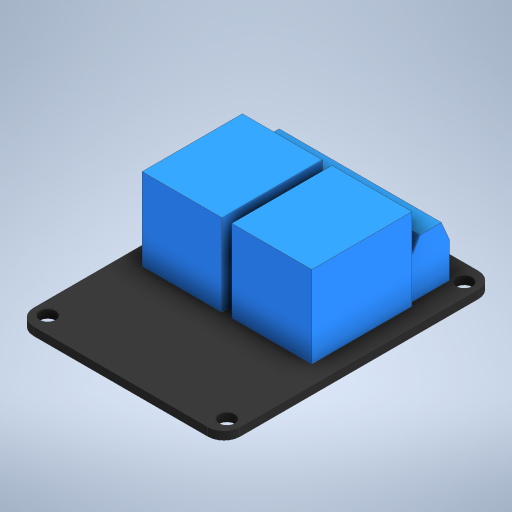
# Autodesk Inventor part: 더블 릴레이 모듈
Saved by Autodesk Inventor 2023.1 (Build 271208000, 208)
## iProperties
Created: 2022-08-14
Part Number: 더블 릴레이 모듈
Material: 일반
Document SubType Name: Modeling
Designer: fly01
Density: 1 g/cm^3
Appearance: 기본값
Author: fly01
Autodesk Inventor part; units mm, degrees
ref_plane "YZ Plane" through (0, 0, 0) normal (1, 0, 0) x (0, 1, 0)
ref_plane "XZ Plane" through (0, 0, 0) normal (0, 1, 0) x (-1, 0, 0)
ref_plane "XY Plane" through (0, 0, 0) normal (0, 0, 1) x (1, 0, 0)
sketch "스케치1" plane through (0, 0, 0) normal (0, 0, 1) x (1, 0, 0)
  point P0 (0, 0)
sketch "스케치2" plane through (0, 0, 0) normal (0, 1, 0) x (-1, 0, 0)
  line L0 (-16.35, -25.35) -> (16.35, -25.35)
  line L1 (19.35, -22.35) -> (19.35, 22.35)
  line L2 (16.35, 25.35) -> (-16.35, 25.35)
  line L3 (-19.35, 22.35) -> (-19.35, -22.35)
  line L4 (-19.35, -25.35) -> (19.35, 25.35) construction
  line L5 (19.35, -25.35) -> (-19.35, 25.35) construction
  circle A0 centre (16.8, 22.25) radius 1.5
  line L6 (0, 0) -> (0, -6.2498)
  line L7 (0, 0) -> (4.685, 0)
  circle A1 centre (16.8, -22.25) radius 1.5
  circle A2 centre (-16.8, 22.25) radius 1.5
  circle A3 centre (-16.8, -22.25) radius 1.5
  arc A4 (19.35, 22.35) -> (16.35, 25.35) centre (16.35, 22.35) ccw
  arc A5 (16.35, -25.35) -> (19.35, -22.35) centre (16.35, -22.35) ccw
  arc A6 (-19.35, -22.35) -> (-16.35, -25.35) centre (-16.35, -22.35) ccw
  arc A7 (-16.35, 25.35) -> (-19.35, 22.35) centre (-16.35, 22.35) ccw
  dimension "d0" = 38.7
  dimension "d1" = 50.7
  dimension "d2" = 3
  dimension "d3" = 30.6
  dimension "d4" = 44.5
  dimension "d5" = 3
  constraints: 16 end point, 8 centre point, 8 point on circle, 8 point on line, 8 tangent, 3 equal radius, 3 symmetric about line, 2 horizontal, 2 midpoint, 2 parallel, 1 perpendicular, 1 vertical, 3 other
  measures "d0" distance of L5.end L4.end
  measures "d1" distance of L4.end L5.start
  measures "d2" diameter of A0
  measures "d4" distance of A3.centre A2.centre
  measures "d5" radius of A4
extrude "돌출1" add sketch "스케치2" along normal blind 1.55
sketch "스케치3" plane through (0, 1.55, 0) normal (0, 1, 0) x (1, 0, 0)
  line L0 (-15.9, -5.45) -> (-0.9, -5.45)
  line L1 (-0.9, -5.45) -> (-0.9, 13.35)
  line L2 (-0.9, 13.35) -> (-15.9, 13.35)
  line L3 (-15.9, 13.35) -> (-15.9, -5.45)
  line L4 (-15.9, -5.45) -> (-0.9, 13.35) construction
  line L5 (-0.9, -5.45) -> (-15.9, 13.35) construction
  line L6 (16.35, 25.35) -> (-16.35, 25.35) projected
  line L7 (0, 0) -> (0, -13.7943)
  line L8 (15.9, -5.45) -> (0.9, -5.45)
  line L9 (0.9, -5.45) -> (0.9, 13.35)
  line L10 (0.9, 13.35) -> (15.9, 13.35)
  line L11 (15.9, 13.35) -> (15.9, -5.45)
  line L12 (15.9, -5.45) -> (0.9, 13.35) construction
  line L13 (0.9, -5.45) -> (15.9, 13.35) construction
  point P0 (-8.4, 3.95)
  point P1 (8.4, 3.95)
  dimension "d8" = 15
  dimension "d9" = 18.8
  dimension "d10" = 0.9
  dimension "d11" = 12
  constraints: 26 end point, 5 symmetric about line, 2 midpoint, 2 parallel, 1 horizontal, 1 perpendicular, 1 vertical
  measures "d8" distance of L2.end L1.end
  measures "d9" distance of L1.end L0.end
  measures "d10" distance from line of L1 L7.start
  measures "d11" distance between parallel lines of L6 L2
extrude "돌출2" add sketch "스케치3" along normal blind 15.4
sketch "스케치4" plane through (0, 0, 0) normal (1, 0, 0) x (0, 1, 0)
  line L0 (1.55, -22.35) -> (1.55, 22.35) projected
  line L1 (11.75, -13.45) -> (1.55, -13.45)
  line L2 (1.55, -13.45) -> (1.55, -21.05)
  line L3 (1.55, -21.05) -> (11.75, -21.05)
  line L4 (11.75, -21.05) -> (11.75, -13.45)
  line L5 (0, -25.35) -> (1.55, -25.35) projected
  line L6 (11.75, -19.55) -> (8.25, -21.05)
  line L7 (1.55, -13.35) -> (16.95, -13.35) projected
  line L8 (8.25, -13.45) -> (11.75, -15.45)
  point P0 (0, 0)
  point P1 (1.55, -13.45)
  dimension "d16" = 7.6
  dimension "d17" = 10.2
  dimension "d18" = 4.3
  dimension "d19" = 1.5
  dimension "d20" = 2
  dimension "d21" = 3.5
  constraints: 12 end point, 5 point on line, 2 parallel, 1 horizontal, 1 perpendicular, 1 vertical alignment
  measures "d16" distance of L3.end L1.start
  measures "d17" distance of L2.end L3.end
  measures "d18" distance between parallel lines of L5 L3
  measures "d19" distance of L3.end L6.start
  measures "d20" distance from line of L1 L8.end
  measures "d21" distance of L3.end L6.end
extrude "돌출3" add sketch "스케치4" along normal mid plane 30.4 contours L0 L1 L8 L4 L6 L3
